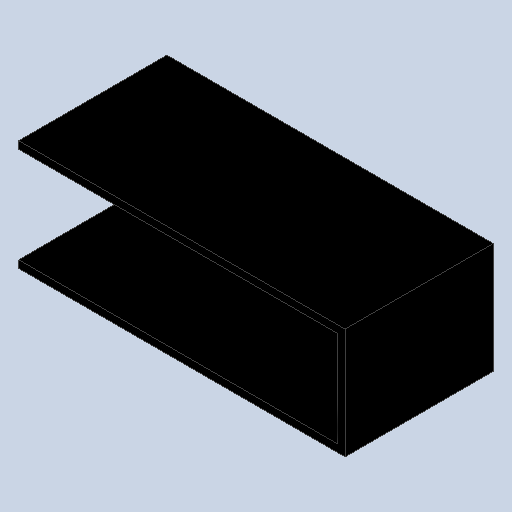
# Autodesk Inventor part: emax box
Saved by Autodesk Inventor 2025.2 (Build 292293000, 293)
## iProperties
Category: <PART CATAGORY>
Created: 2025-01-15
Part Number: emax box
Material: Generic
Document SubType Name: Modeling
Designer: lachl
Density: 1 g/cm^3
Appearance: Default
Title: <TITLE>
Author: lachl
Revision Number: 1
Autodesk Inventor part; units mm, degrees
ref_plane "YZ Plane" through (0, 0, 0) normal (1, 0, 0) x (0, 1, 0)
ref_plane "XZ Plane" through (0, 0, 0) normal (0, 1, 0) x (-1, 0, 0)
ref_plane "XY Plane" through (0, 0, 0) normal (0, 0, 1) x (1, 0, 0)
sketch "Sketch6" plane through (0, 0, 0) normal (0, 0, 1) x (1, 0, 0)
  line L0 (-12.4, 5.9) -> (12.4, 5.9)
  line L1 (12.4, 5.9) -> (12.4, -5.9)
  line L2 (12.4, -5.9) -> (-12.4, -5.9)
  line L3 (-12.4, -5.9) -> (-12.4, 5.9)
  point P0 (0, 0)
  point P1 (-12.4, 0)
  point P2 (0, 5.9)
  dimension "d85" = 11.8
  dimension "d86" = 24.8
  constraints: 8 end point, 2 midpoint, 2 parallel, 1 horizontal, 1 horizontal alignment, 1 perpendicular, 1 vertical alignment
  measures "d85" distance of L2.end L0.start
  measures "d86" distance of L0.start L0.end
extrude "Extrusion3" add sketch "Sketch6" along normal blind 0.8
sketch "Sketch7" plane through (0, 0, 0.8) normal (0, 0, 1) x (1, 0, 0)
  point P0 (0, 0)
sketch "Sketch8" plane through (0, 0, 0.8) normal (0, 0, 1) x (1, 0, 0)
  line L0 (12.4, 5.9) -> (-12.4, 5.9) projected
  line L1 (-12.4, -5.9) -> (12.4, -5.9) projected
  line L2 (-12.4, 5.9) -> (-10.5276, 5.9)
  line L3 (-10.5276, -5.9) -> (-12.4, -5.9)
  line L4 (-12.4, -5.9) -> (-12.4, 5.9)
  line L5 (12.4, -5.9) -> (-10.5276, -5.9)
  line L6 (12.4163, 5.9) -> (10.7456, 5.9)
  line L7 (-12.4, 5.1) -> (11.6, 5.1)
  line L8 (11.6, 5.1) -> (11.6, -5.1)
  line L9 (11.6, -5.1) -> (-12.4, -5.1)
  line L10 (12.4, -5.9) -> (12.4, 5.9) projected
  point P0 (0, 0)
  dimension "d89" = 0.8
  dimension "d91" = 0.8
  dimension "d92" = 0.8
  constraints: 16 end point, 4 horizontal, 4 point on line, 3 perpendicular, 2 parallel
  measures "d89" distance between parallel lines of L0 L7
  measures "d91" distance between parallel lines of L1 L9
  measures "d92" distance between parallel lines of L10 L8
extrude "Extrusion4" add sketch "Sketch8" along normal blind 15 contours L10 L1 L4 L9 L8 L7 L0
sketch "Sketch9" plane through (-12.4, -5.9, 0) normal (-1, 0, 0) x (0, 0, 1)
  line L0 (0, 11.8) -> (15.8, 11.8) projected
  line L1 (0.8, 11) -> (15.8, 11) projected
  line L2 (15.8, 11.8) -> (15.8, 11)
  line L3 (15.8, 11) -> (0.8, 11)
  line L4 (0.8, 0.8) -> (15.8, 0.8) projected
  line L5 (0.8, 11) -> (0.8, 0.8)
  line L6 (0.8, 0.8) -> (15.8, 0.8)
  line L7 (0, 0) -> (15.8, 0) projected
  line L8 (15.8, 0.8) -> (15.8, 0)
  line L9 (15.8, 0) -> (0, 0)
  line L10 (0, 0) -> (0, 11.8)
  line L11 (0, 11.8) -> (15.8, 11.8)
  point P0 (0, 5.9)
  dimension "d95" = 0.8
  constraints: 16 end point, 6 perpendicular, 2 collinear
  measures "d95" distance of L4.end L7.end
extrude "Extrusion5" add sketch "Sketch9" along normal blind 10
body "Solid2"
